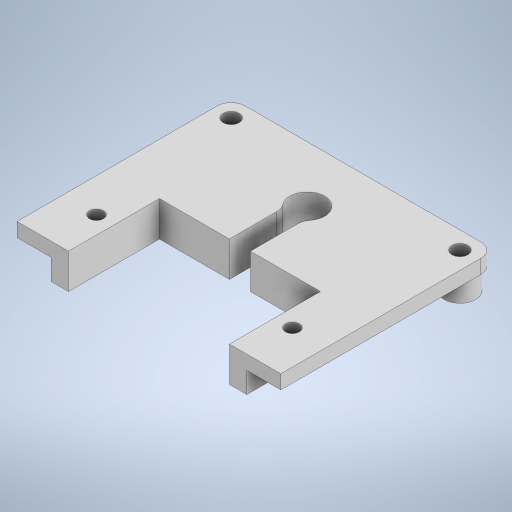
# Autodesk Inventor part: ServoFullMountInsert
Saved by Autodesk Inventor 2024 (Build 280153000, 153)
## iProperties
Created: 2024-04-03
Part Number: ServoFullMountInsert
Material: Generic
Document SubType Name: Modeling
Designer: ringl
Density: 1 g/cm^3
Appearance: Default
Author: ringl
Autodesk Inventor part; units mm, degrees
ref_plane "YZ Plane" through (0, 0, 0) normal (1, 0, 0) x (0, 1, 0)
ref_plane "XZ Plane" through (0, 0, 0) normal (0, 1, 0) x (-1, 0, 0)
ref_plane "XY Plane" through (0, 0, 0) normal (0, 0, 1) x (1, 0, 0)
sketch "Sketch1" plane through (0, 0, 0) normal (0, 1, 0) x (-1, 0, 0)
  line L0 (0, 0) -> (28, 0)
  line L1 (28, 0) -> (28, -38.5)
  line L2 (28, -38.5) -> (0, -38.5)
  line L3 (0, -38.5) -> (0, 0)
  dimension "d0" = 28
  dimension "d1" = 38.5
  constraints: 8 end point, 2 parallel, 1 horizontal, 1 perpendicular
  measures "d0" distance of L1.end L2.end
  measures "d1" distance of L0.end L1.end
extrude "Extrusion1" add sketch "Sketch1" along normal blind 3
sketch "Sketch2" plane through (0, 3, 0) normal (0, 1, 0) x (1, 0, 0)
  line L0 (-28, 0) -> (0, 0) projected
  circle A0 centre (0, 0) radius 2
  circle A1 centre (-28, 0) radius 2
  line L1 (0, 38.5) -> (-28, 38.5) projected
  circle A2 centre (-28, 38.5) radius 2
  circle A3 centre (0, 38.5) radius 2
  dimension "d8" = 4
  dimension "d9" = 4
  dimension "d10" = 4
  dimension "d11" = 4
  constraints: 4 centre point, 3 coincident
  measures "d8" diameter of A0
  measures "d9" diameter of A1
  measures "d10" diameter of A2
  measures "d11" diameter of A3
extrude "Extrusion2" cut sketch "Sketch2" against normal blind 3
sketch "Sketch3" plane through (0, 3, 0) normal (0, 1, 0) x (1, 0, 0)
  line L0 (-32.85, 43.35) -> (4.85, 43.35)
  line L1 (4.85, 43.35) -> (4.85, -4.85)
  line L2 (4.85, -4.85) -> (-32.85, -4.85)
  line L3 (-32.85, -4.85) -> (-32.85, 43.35)
  line L4 (-2, 38.5) -> (-26, 38.5) projected
  line L5 (0, 2) -> (0, 36.5) projected
  point P0 (0, 0)
  point P1 (-2, 6.25)
  point P2 (-26, 32.25)
  dimension "d14" = 48.2
  dimension "d15" = 37.7
  dimension "d16" = 4.85
  dimension "d17" = 4.85
  constraints: 8 end point, 2 parallel, 1 horizontal, 1 perpendicular
  measures "d14" distance of L0.end L1.end
  measures "d15" distance of L1.end L2.end
  measures "d16" distance between parallel lines of L0 L4
  measures "d17" distance between parallel lines of L5 L1
extrude "Extrusion3" add sketch "Sketch3" along normal blind 2
sketch "Sketch4" plane through (0, 3, 0) normal (0, -1, 0) x (1, 0, 0)
  circle A0 centre (2.35, -40.85) radius 2.25
  line L0 (-2, -38.5) -> (-26, -38.5) projected
  line L1 (0, -2) -> (0, -36.5) projected
  circle A1 centre (-30.35, -40.85) radius 2.25
  line L2 (-28, -36.5) -> (-28, -2) projected
  circle A2 centre (-30.35, 2.35) radius 2.25
  line L3 (-26, 0) -> (-2, 0) projected
  circle A3 centre (2.35, 2.35) radius 2.25
  point P0 (0, 0)
  dimension "d20" = 4.5
  dimension "d21" = 2.35
  dimension "d22" = 2.35
  dimension "d23" = 4.5
  dimension "d24" = 2.35
  dimension "d25" = 2.35
  dimension "d26" = 4.5
  dimension "d27" = 2.35
  dimension "d28" = 4.5
  dimension "d29" = 2.35
  dimension "d30" = 2.35
  dimension "d31" = 2.35
  constraints: 4 centre point
  measures "d20" diameter of A0
  measures "d21" distance from line of A0.centre L0
  measures "d22" distance from line of A0.centre L1
  measures "d23" diameter of A1
  measures "d24" distance from line of L2 A1.centre
  measures "d25" distance from line of L0 A1.centre
  measures "d26" diameter of A2
  measures "d27" distance from line of L3 A2.centre
  measures "d28" diameter of A3
  measures "d29" distance from line of L1 A3.centre
  measures "d30" distance from line of L3 A3.centre
  measures "d31" distance from line of L2 A2.centre
extrude "Extrusion4" add sketch "Sketch4" along normal blind 3
fillet "Fillet1" radius 2 4 edges at (4.85, 4, -43.35) (4.85, 4, 4.85) (-32.85, 4, 4.85) (-32.85, 4, -43.35)
sketch "Sketch5" plane through (0, 5, 0) normal (0, 1, 0) x (1, 0, 0)
  circle A0 centre (0, 19.25) radius 1
  circle A1 centre (-28, 19.25) radius 1
  line L0 (4.85, -2.85) -> (4.85, 41.35) projected
  line L1 (-30.85, -4.85) -> (2.85, -4.85) projected
  point P0 (0, 0)
  dimension "d45" = 2
  dimension "d46" = 2
  dimension "d73" = 28
  dimension "d81" = 24.1
  dimension "d82" = 4.85
  constraints: 2 centre point, 1 horizontal alignment
  measures "d45" diameter of A0
  measures "d46" diameter of A1
  measures "d73" distance of A1.centre A0.centre
  measures "d81" distance from line of L1 A0.centre
  measures "d82" distance from line of L0 A0.centre
extrude "Extrusion6" cut sketch "Sketch5" against normal through all
sketch "Sketch8" plane through (0, 5, 0) normal (0, 1, 0) x (1, 0, 0)
  circle A0 centre (-14, 3.125) radius 1.75
  line L0 (-2, 6.25) -> (-26, 6.25) projected
  line L1 (-26, 0) -> (-2, 0) projected
  line L2 (-32.85, 41.35) -> (-32.85, -2.85) projected
  point P0 (0, 0)
  dimension "d68" = 3.5
  dimension "d69" = 3.125
  dimension "d70" = 18.85
  constraints: 1 centre point
  measures "d68" diameter of A0
  measures "d69" distance from line of L1 A0.centre
  measures "d70" distance from line of L2 A0.centre
extrude "Extrusion9" cut sketch "Sketch8" against normal through all
sketch "Sketch9" plane through (0, 5, 0) normal (0, 1, 0) x (1, 0, 0)
  circle A0 centre (-14, 3.125) radius 1.75 projected
  line L0 (-15, 4.5611) -> (-15, 6.25)
  line L1 (-15, 6.25) -> (-13, 6.25)
  line L2 (-13, 6.25) -> (-13, 4.5611)
  arc A1 (-13, 4.5611) -> (-15, 4.5611) centre (-14, 3.125) ccw
  line L3 (-2, 6.25) -> (-26, 6.25) projected
  point P0 (0, 0)
  point P1 (-14, 6.25)
  dimension "d76" = 2
  dimension "d77" = 1
  constraints: 6 end point, 4 point on circle, 2 midpoint, 2 perpendicular, 1 centre point, 1 concentric, 1 vertical
  measures "d76" distance of L0.end L1.end
  measures "d77" distance from line of A0.centre L2
extrude "Extrusion10" cut sketch "Sketch9" against normal through all contours A0 L0 L1 L2
fillet "Fillet2" radius 2 2 edges at (-15, 2.5, -4.5611) (-13, 2.5, -4.5611)
sketch "Sketch10" plane through (0, 5, 0) normal (0, 1, 0) x (1, 0, 0)
  line L0 (-25.5, 12.75) -> (-2.5, 12.75)
  line L1 (-2.5, 12.75) -> (-2.5, 25.75)
  line L2 (-2.5, 25.75) -> (-25.5, 25.75)
  line L3 (-25.5, 25.75) -> (-25.5, 12.75)
  line L4 (-32.85, 41.35) -> (-32.85, -2.85) projected
  circle A0 centre (-28, 19.25) radius 1 projected
  point P0 (0, 0)
  dimension "d83" = 23
  dimension "d84" = 13
  dimension "d85" = 7.35
  dimension "d86" = 6.5
  constraints: 8 end point, 2 parallel, 1 horizontal, 1 perpendicular
  measures "d83" distance of L2.end L1.end
  measures "d84" distance of L1.end L0.end
  measures "d85" distance between parallel lines of L4 L3
  measures "d86" distance from line of L2 A0.centre
extrude "Extrusion11" cut sketch "Sketch10" against normal through all contours L3 L2 L1 L0
sketch "Sketch11" plane through (0, 5, 0) normal (0, 1, 0) x (1, 0, 0)
  line L0 (4.85, -4.85) -> (-32.85, -4.85)
  line L1 (-32.85, -4.85) -> (-32.85, 12.75)
  line L2 (-32.85, 12.75) -> (4.85, 12.75)
  line L3 (4.85, 12.75) -> (4.85, -4.85)
  line L4 (-2.5, 12.75) -> (-25.5, 12.75) projected
  point P0 (0, 0)
  point P1 (-32.85, -2.85)
  point P2 (2.85, -4.85)
  point P3 (4.85, -2.85)
  constraints: 8 end point, 4 point on line, 2 parallel, 1 horizontal, 1 perpendicular
extrude "Extrusion12" cut sketch "Sketch11" against normal through all
sketch "Sketch12" plane through (0, 5, 0) normal (0, 1, 0) x (1, 0, 0)
  circle A0 centre (-14, 35.375) radius 2.5
  line L0 (-2, 38.5) -> (-26, 38.5) projected
  line L1 (4.85, 12.75) -> (4.85, 41.35) projected
  point P0 (0, 0)
  point P1 (-14, 38.5)
  dimension "d92" = 5
  dimension "d93" = 3.125
  dimension "d94" = 18.85
  constraints: 1 centre point, 1 midpoint
  measures "d92" diameter of A0
  measures "d93" distance of point (-14, 38.5) A0.centre
  measures "d94" distance from line of L1 A0.centre
extrude "Extrusion13" cut sketch "Sketch12" against normal through all
sketch "Sketch13" plane through (0, 5, 0) normal (0, 1, 0) x (1, 0, 0)
  circle A0 centre (-14, 35.375) radius 2.5 projected
  line L0 (-15.5, 33.375) -> (-15.5, 25.75)
  line L1 (-2.5, 25.75) -> (-25.5, 25.75) projected
  line L2 (-12.5, 33.375) -> (-12.5, 19.264)
  point P0 (0, 0)
  point P1 (-12.5, 25.75)
  dimension "d97" = 3
  constraints: 4 end point, 2 point on circle, 2 vertical, 1 horizontal alignment, 1 point on line
  measures "d97" distance between parallel lines of L2 L0
extrude "Extrusion14" cut sketch "Sketch13" against normal through all contours A0 L2 L1 L0
fillet "Fillet3" radius 2 2 edges at (-12.5, 2.5, -33.375) (-15.5, 2.5, -33.375)
sketch "Sketch14" plane through (-30.35, 0, -40.85) normal (0, -1, 0) x (1, 0, 0)
  circle A0 centre (32.7, 0) radius 2.25 projected
  circle A1 centre (0, 0) radius 2.25 projected
  circle A2 centre (32.7, 0) radius 1.15
  circle A3 centre (0, 0) radius 1.15
  point P0 (30.35, 40.85)
  dimension "d101" = 2.3
  dimension "d102" = 2.3
  constraints: 2 centre point, 2 coincident
  measures "d101" diameter of A2
  measures "d102" diameter of A3
extrude "Extrusion15" cut sketch "Sketch14" against normal through all contours A2 | A3
body "Solid1"
